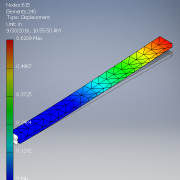
# Autodesk Inventor part: test bar
Saved by Autodesk Inventor 2017 (Build 210142000, 142)
## iProperties
Created: 2016-09-30
Part Number: test bar
Material: Bronze, Cast
Document SubType Name: Modeling
Designer: canti021
Density: 8.87 g/cm^3
Appearance: Bronze - Satin
Author: canti021
Autodesk Inventor part; units mm, degrees
ref_plane "YZ Plane" through (0, 0, 0) normal (1, 0, 0) x (0, 1, 0)
ref_plane "XZ Plane" through (0, 0, 0) normal (0, 1, 0) x (-1, 0, 0)
ref_plane "XY Plane" through (0, 0, 0) normal (0, 0, 1) x (1, 0, 0)
sketch "Sketch1" plane through (0, 0, 0) normal (0, 0, 1) x (1, 0, 0)
  line L0 (-1.5875, 0) -> (23.8125, 0)
  line L1 (23.8125, 0) -> (23.8125, -6.35)
  line L2 (23.8125, -6.35) -> (-1.5875, -6.35)
  line L3 (-1.5875, -6.35) -> (-1.5875, 0)
  point P0 (0, 0)
  constraints: 8 end point, 2 parallel, 1 horizontal, 1 perpendicular
extrude "Extrusion1" add sketch "Sketch1" along normal blind 314.325
body "Solid1"
